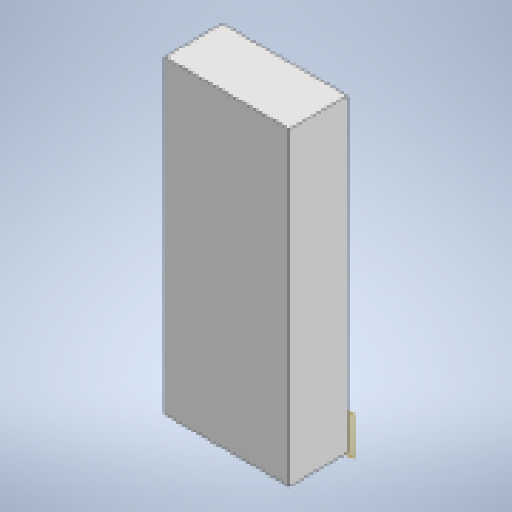
# Autodesk Inventor part: _hand_2_
Saved by Autodesk Inventor 2024.3 (Build 283343000, 343)
## iProperties
Created: 2024-09-06
Part Number: _hand_2_
Material: 일반
Document SubType Name: Modeling
Designer: gretc
Density: 1 g/cm^3
Appearance: 기본값
Author: gretc
Autodesk Inventor part; units mm, degrees
ref_plane "YZ Plane" through (0, 0, 0) normal (1, 0, 0) x (0, 1, 0)
ref_plane "XZ Plane" through (0, 0, 0) normal (0, 1, 0) x (-1, 0, 0)
ref_plane "XY Plane" through (0, 0, 0) normal (0, 0, 1) x (1, 0, 0)
ref_plane "작업 평면1" through (0, 0, 0) normal (0, 0, 1) x (1, 0, 0)
sketch "스케치1" plane through (0, 0, 0) normal (0, 0, 1) x (1, 0, 0)
  line L0 (0, 0) -> (21.6, 0) projected
  line L1 (21.6, 0) -> (21.6, 6) projected
  line L2 (0, 6) -> (21.6, 6) projected
  line L3 (0, 0) -> (0, 6) projected
  line L4 (0, 47.5) -> (21.6, 47.5) projected
  line L5 (21.6, 47.5) -> (21.6, 53.5) projected
  line L6 (0, 53.5) -> (21.6, 53.5) projected
  line L7 (0, 47.5) -> (0, 53.5) projected
  line L8 (0, 0) -> (21.6, 0)
  line L9 (21.6, 0) -> (21.6, 53.5)
  line L10 (21.6, 53.5) -> (0, 53.5)
  line L11 (0, 53.5) -> (0, 0)
  constraints: 8 end point, 2 parallel, 1 horizontal, 1 perpendicular
ref_plane "작업 평면2" through (0, 0, 0) normal (0, 0, 1) x (1, 0, 0)
sketch "스케치2" plane through (0, 0, 0) normal (0, 0, 1) x (1, 0, 0)
  point P0 (0, 0)
extrude "돌출1" add sketch "스케치1" along normal blind 10
